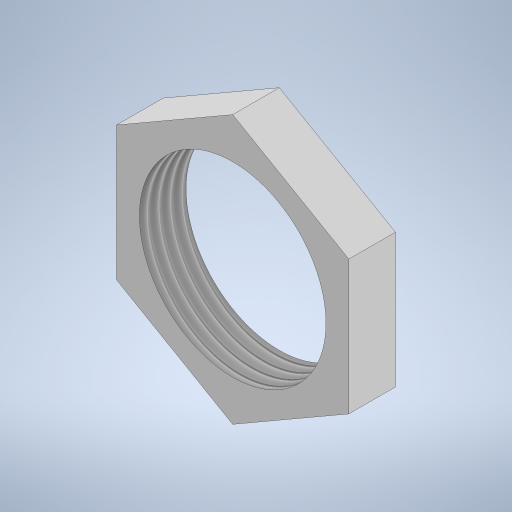
# Autodesk Inventor part: Деталь2
Saved by Autodesk Inventor 2023.1 (Build 271208000, 208)
## iProperties
Created: 2025-08-10
Part Number: Деталь2
Material: Типовые
Document SubType Name: Modeling
Designer: DELL
Density: 1 g/cm^3
Appearance: По умолчанию
Author: DELL
Autodesk Inventor part; units mm, degrees
ref_plane "YZ Plane" through (0, 0, 0) normal (1, 0, 0) x (0, 1, 0)
ref_plane "XZ Plane" through (0, 0, 0) normal (0, 1, 0) x (-1, 0, 0)
ref_plane "XY Plane" through (0, 0, 0) normal (0, 0, 1) x (1, 0, 0)
sketch "Эскиз1" plane through (0, 0, 0) normal (0, 0, 1) x (1, 0, 0)
  line L0 (0, -23) -> (-19.9186, -11.5)
  line L1 (-19.9186, -11.5) -> (-19.9186, 11.5)
  line L2 (-19.9186, 11.5) -> (0, 23)
  line L3 (0, 23) -> (19.9186, 11.5)
  line L4 (19.9186, 11.5) -> (19.9186, -11.5)
  line L5 (19.9186, -11.5) -> (0, -23)
  circle A0 centre (0, 0) radius 16
  dimension "d1" = 32
  dimension "d3" = 46
  constraints: 12 end point, 2 coincident, 1 centre point, 13 other
  measures "d1" diameter of A0
  measures "d3" distance of L0.start L2.end
extrude "Выдавливание1" add sketch "Эскиз1" along normal blind 8
thread "Резьба1" size "M32x2" class "6H" standard "ANSI Metric M Profile" length 60
